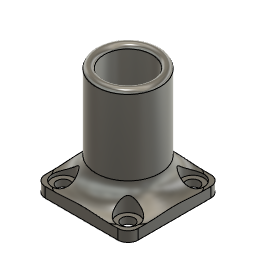
Landing Gear Mounts v4 (Autodesk Fusion 360 design; units mm, degrees)
Autodesk Fusion 360 part; units mm, degrees
sketch "Sketch1" plane through (0, 0, 0) normal (0, 1, 0) x (1, 0, 0)
  line L0 (0, 0) -> (23, 0)
  line L1 (23, 0) -> (23, 23)
  line L2 (23, 23) -> (0, 23)
  line L3 (0, 23) -> (0, 0)
  circle A0 centre (3.5, 19.5) radius 1.6
  line L4 (0, 0) -> (0, 11.5) construction
  line L5 (0, 23) -> (11.5, 23) construction
  circle A1 centre (19.5, 19.5) radius 1.6
  circle A2 centre (3.5, 3.5) radius 1.6
  circle A3 centre (19.5, 3.5) radius 1.6
  dimension "d1" = 23
  dimension "d2" = 23
  dimension "d3" = 3.2
  dimension "d4" = 11.5
  dimension "d5" = 8
  dimension "d6" = 11.5
  dimension "d7" = 8
  dimension "d13" = 16
  dimension "d14" = -16
  constraint horizontal L0
  constraint vertical L1
  constraint horizontal L2
  constraint vertical L3
  constraint coincident L0.start L3.end
  constraint perpendicular L0 L4
  constraint perpendicular L3 L5
  measures "d1" distance of L0.start L0.end
  measures "d2" distance of L0.start L2.end
  measures "d3" diameter of A0
  measures "d4" distance of L0.start L4.end
  measures "d5" vertical distance of A0.centre L4.end
  measures "d6" distance of L2.end L5.end
  measures "d7" horizontal distance of A0.centre L5.end
extrude "Extrude1" add sketch "Sketch1" along normal blind 2.5
fillet "Fillet1" radius 2.5 4 edges at (0, 1.25, 0) (23, 1.25, 0) (23, 1.25, -23) (0, 1.25, -23)
sketch "Sketch2" plane through (0, 2.5, 0) normal (0, 1, 0) x (-1, 0, 0)
  arc A0 (-2.5, -23) -> (0, -20.5) centre (-2.5, -20.5) ccw
  line L0 (0, -20.5) -> (0, -2.5)
  arc A1 (0, -2.5) -> (-2.5, 0) centre (-2.5, -2.5) ccw
  line L1 (-2.5, 0) -> (-20.5, 0)
  arc A2 (-20.5, 0) -> (-23, -2.5) centre (-20.5, -2.5) ccw
  line L2 (-23, -2.5) -> (-23, -20.5)
  arc A3 (-23, -20.5) -> (-20.5, -23) centre (-20.5, -20.5) ccw
  line L3 (-20.5, -23) -> (-2.5, -23)
  circle A4 centre (-19.5, -19.5) radius 1.6
  circle A5 centre (-19.5, -3.5) radius 1.6
  circle A6 centre (-3.5, -3.5) radius 1.6
  circle A7 centre (-3.5, -19.5) radius 1.6
  circle A8 centre (-3.5, -19.5) radius 2.75
  circle A9 centre (-19.5, -19.5) radius 2.75
  circle A10 centre (-3.5, -3.5) radius 2.75
  circle A11 centre (-19.5, -3.5) radius 2.75
  dimension "d19" = 5.5
  dimension "d20" = 5.5
  dimension "d21" = 5.5
  dimension "d22" = 5.5
  constraint concentric A7 A8
  constraint concentric A4 A9
  constraint concentric A6 A10
  constraint concentric A5 A11
  measures "d19" diameter of A8
  measures "d20" diameter of A9
  measures "d21" diameter of A10
  measures "d22" diameter of A11
extrude "Extrude2" cut sketch "Sketch2" against normal blind 0.8 contours A8 | A9 | A10 | A11
sketch "Sketch3" plane through (0, 2.5, 0) normal (0, 1, 0) x (-1, 0, 0)
  circle A0 centre (-19.5, -19.5) radius 2.75
  circle A1 centre (-3.5, -3.5) radius 2.75
  circle A2 centre (-3.5, -19.5) radius 2.75
  circle A3 centre (-19.5, -3.5) radius 2.75
  arc A4 (-2.5, -23) -> (0, -20.5) centre (-2.5, -20.5) ccw
  line L0 (0, -20.5) -> (0, -2.5)
  arc A5 (0, -2.5) -> (-2.5, 0) centre (-2.5, -2.5) ccw
  line L1 (-2.5, 0) -> (-20.5, 0)
  arc A6 (-20.5, 0) -> (-23, -2.5) centre (-20.5, -2.5) ccw
  line L2 (-23, -2.5) -> (-23, -20.5)
  arc A7 (-23, -20.5) -> (-20.5, -23) centre (-20.5, -20.5) ccw
  line L3 (-20.5, -23) -> (-2.5, -23)
  circle A8 centre (-11.5, -11.5) radius 5.9
  circle A9 centre (-11.5, -11.5) radius 7.9
  dimension "d25" = 11.8
  dimension "d26" = 11.5
  dimension "d27" = 11.5
  dimension "d28" = 15.8
  constraint concentric A8 A9
  measures "d25" diameter of A8
  measures "d26" distance of L0 A8.centre
  measures "d27" distance of L1 A8.centre
  measures "d28" diameter of A9
extrude "Extrude3" add sketch "Sketch3" along normal blind 25 contours A9
fillet "Fillet2" radius 5.5 1 edges at (18.8654, 2.5, -8.6432)
fillet "Fillet3" radius 1 2 edges at (18.8654, 27.5, -14.3568) (17.0007, 27.5, -9.3665)
sketch "Sketch4" plane through (0, 0, 0) normal (1, 0, 0) x (0, 0, -1)
equation "d4 = ( 23 / 2 ) * 1 mm"
equation "d5 = ( 16 / 2 ) * 1 mm"
equation "d28 = 11.8 mm + 4 mm"
